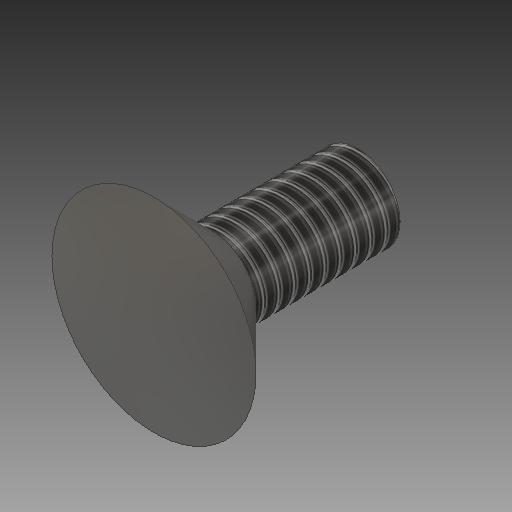
# Autodesk Inventor part: ネジ皿m4,08
Saved by Autodesk Inventor 2020 (Build 240168000, 168)
## iProperties
Part Number: ネジ皿m4,08
Material: 鋼、高強度、低合金
Document SubType Name: Modeling
Designer: 雪村
Density: 7.85 g/cm^3
Appearance: 鋼 - つや出し
Mass: 0.868428 g
Surface Area: 1.76684 cm^2
Volume: 0.110628 cm^3
Author: 雪村
Autodesk Inventor part; units mm, degrees
ref_plane "YZ Plane" through (0, 0, 0) normal (1, 0, 0) x (0, 1, 0)
ref_plane "XZ Plane" through (0, 0, 0) normal (0, 1, 0) x (-1, 0, 0)
ref_plane "XY Plane" through (0, 0, 0) normal (0, 0, 1) x (1, 0, 0)
sketch "スケッチ1" plane through (0, 0, 0) normal (0, 0, 1) x (1, 0, 0)
  circle A0 centre (0, 0) radius 1.65
  dimension "d0" = 3.3
  constraints: 1 centre point, 1 coincident
  measures "d0" diameter of A0
extrude "押し出し1" add sketch "スケッチ1" along normal blind 8
sketch "スケッチ2" plane through (0, 0, 8) normal (0, 0, 1) x (1, 0, 0)
  circle A0 centre (0, 0) radius 4
  dimension "d3" = 8
  constraints: 1 centre point, 1 coincident
  measures "d3" diameter of A0
extrude "押し出し2" add sketch "スケッチ2" against normal blind 2.3
chamfer "面取り1" distance 2.3 angle 45 1 edges at (-4, 0, 5.7)
thread "ねじ1" size "M3.5x0.6" class "6g" standard "ANSI Metric M Profile" full length
